Autodesk Inventor part; units mm, degrees
(part 6 of 6)
sketch "Sketch77" plane through (-67.6485, -56.3001, 10) normal (0, 0, -1) x (-1, 0, 0)
  line L0 (26.7044, 28.81) -> (18.3959, 20.5015)
  arc A0 (17.4062, 16.708) -> (18.3959, 20.5015) centre (3.9071, 22.2557) ccw
  line L1 (17.4062, 16.708) -> (10.5397, 0)
  line L2 (10.5397, 0) -> (0, 0)
  line L3 (0, 0) -> (0, -30)
  line L4 (0, -30) -> (10.5397, -30)
  line L5 (10.5397, -30) -> (17.4062, -46.708)
  arc A1 (18.3959, -50.5015) -> (17.4062, -46.708) centre (3.9071, -52.2557) ccw
  line L6 (18.3959, -50.5015) -> (26.7044, -58.81)
  line L7 (8.6997, -15) -> (26.7044, -58.81)
  line L8 (26.7044, 28.81) -> (8.6997, -15)
  line L9 (8.034, -77.4804) -> (-6.8327, -62.6138)
  line L10 (-6.8327, -62.6138) -> (-8.2078, -61.6851)
  line L11 (-8.2078, -61.6851) -> (-8.5835, -61.4603)
  line L12 (-8.5835, -61.4603) -> (-27.5835, -51.4603)
  line L13 (-27.5835, -51.4603) -> (-31.3094, -51.4603)
  line L14 (-31.3094, -51.4603) -> (-50.3094, -61.4603)
  line L15 (-50.3094, -61.4603) -> (-52.2336, -63.7126)
  line L16 (-52.2336, -63.7126) -> (-53.8304, -68.4099)
  arc A2 (-54.4465, -69.9343) -> (-53.8304, -68.4099) centre (-67.6485, -63.7126) ccw
  line L17 (-54.4465, -69.9343) -> (-54.4465, -82.65)
  line L18 (-48.4465, -65) -> (-54.4465, -82.65)
  line L19 (-29.4465, -55) -> (-48.4465, -65)
  line L20 (-10.4465, -65) -> (-29.4465, -55)
  line L21 (8.034, -77.4804) -> (-10.4465, -65)
  line L22 (-128.4643, -62.6138) -> (-143.3309, -77.4804)
  line L23 (-124.8505, -65) -> (-143.3309, -77.4804)
  line L24 (-105.8505, -55) -> (-124.8505, -65)
  line L25 (-86.8505, -65) -> (-105.8505, -55)
  line L26 (-80.8505, -82.65) -> (-86.8505, -65)
  line L27 (-80.8505, -82.65) -> (-80.8505, -69.9343)
  arc A3 (-81.4665, -68.4099) -> (-80.8505, -69.9343) centre (-67.6485, -63.7126) ccw
  line L28 (-81.4665, -68.4099) -> (-83.0633, -63.7126)
  line L29 (-83.0633, -63.7126) -> (-84.9875, -61.4603)
  line L30 (-84.9875, -61.4603) -> (-103.9875, -51.4603)
  line L31 (-103.9875, -51.4603) -> (-107.7134, -51.4603)
  line L32 (-107.7134, -51.4603) -> (-126.7134, -61.4603)
  line L33 (-126.7134, -61.4603) -> (-127.0891, -61.6851)
  line L34 (-127.0891, -61.6851) -> (-128.4643, -62.6138)
  line L35 (-50.3094, 31.4603) -> (-31.3094, 21.4603)
  line L36 (-6.8327, 32.6138) -> (8.034, 47.4804)
  line L37 (-10.4465, 35) -> (8.034, 47.4804)
  line L38 (-29.4465, 25) -> (-10.4465, 35)
  line L39 (-48.4465, 35) -> (-29.4465, 25)
  line L40 (-54.4465, 52.65) -> (-48.4465, 35)
  line L41 (-54.4465, 52.65) -> (-54.4465, 39.9343)
  arc A4 (-53.8304, 38.4099) -> (-54.4465, 39.9343) centre (-67.6485, 33.7126) ccw
  line L42 (-53.8304, 38.4099) -> (-52.2336, 33.7126)
  line L43 (-52.2336, 33.7126) -> (-50.3094, 31.4603)
  line L44 (-50.3094, 31.4603) -> (-31.3094, 21.4603)
  line L45 (-31.3094, 21.4603) -> (-27.5835, 21.4603)
  line L46 (-27.5835, 21.4603) -> (-8.5835, 31.4603)
  line L47 (-8.5835, 31.4603) -> (-8.2078, 31.6851)
  line L48 (-8.2078, 31.6851) -> (-6.8327, 32.6138)
  line L49 (-143.3309, 47.4804) -> (-128.4643, 32.6138)
  line L50 (-128.4643, 32.6138) -> (-127.0891, 31.6851)
  line L51 (-127.0891, 31.6851) -> (-126.7134, 31.4603)
  line L52 (-126.7134, 31.4603) -> (-107.7134, 21.4603)
  line L53 (-107.7134, 21.4603) -> (-103.9875, 21.4603)
  line L54 (-103.9875, 21.4603) -> (-84.9875, 31.4603)
  line L55 (-84.9875, 31.4603) -> (-83.0633, 33.7126)
  line L56 (-83.0633, 33.7126) -> (-81.4665, 38.4099)
  arc A5 (-80.8505, 39.9343) -> (-81.4665, 38.4099) centre (-67.6485, 33.7126) ccw
  line L57 (-80.8505, 39.9343) -> (-80.8505, 52.65)
  line L58 (-86.8505, 35) -> (-80.8505, 52.65)
  line L59 (-105.8505, 25) -> (-86.8505, 35)
  line L60 (-124.8505, 35) -> (-105.8505, 25)
  line L61 (-143.3309, 47.4804) -> (-124.8505, 35)
  line L62 (-162.0013, -58.81) -> (-155.7371, -52.5457)
  arc A6 (-155.2161, -49.5915) -> (-155.7371, -52.5457) centre (-141.1799, -53.5901) ccw
  line L63 (-155.2161, -49.5915) -> (-154.2755, -46.2898)
  line L64 (-154.2755, -46.2898) -> (-150.5441, -47.3528)
  line L65 (-150.5441, -47.3528) -> (-144.5534, -41.3621)
  line L66 (-144.5534, -41.3621) -> (-144.3898, -40.7877)
  line L67 (-144.3898, -40.7877) -> (-152.0837, -38.5959)
  line L68 (-152.0837, -38.5959) -> (-151.9306, -37.5)
  line L69 (-151.9306, -37.5) -> (-155.9306, -37.5)
  line L70 (-162.0013, -58.81) -> (-155.9306, -37.5)
  line L71 (-144.5534, 11.3621) -> (-150.5441, 17.3528)
  line L72 (-150.5441, 17.3528) -> (-154.2755, 16.2898)
  line L73 (-154.2755, 16.2898) -> (-155.2161, 19.5915)
  arc A7 (-155.7371, 22.5457) -> (-155.2161, 19.5915) centre (-141.1799, 23.5901) ccw
  line L74 (-155.7371, 22.5457) -> (-162.0013, 28.81)
  line L75 (-155.9306, 7.5) -> (-162.0013, 28.81)
  line L76 (-155.9306, 7.5) -> (-151.9306, 7.5)
  line L77 (-151.9306, 7.5) -> (-152.0837, 8.5959)
  line L78 (-152.0837, 8.5959) -> (-144.3898, 10.7877)
  line L79 (-144.3898, 10.7877) -> (-144.5534, 11.3621)
  arc A8 (26.7044, -58.81) -> (8.034, -77.4804) centre (40.2898, -91.0658) ccw
  arc A9 (-54.4465, -82.65) -> (-80.8505, -82.65) centre (-67.6485, -115.0647) ccw
  arc A10 (-143.3309, -77.4804) -> (-162.0013, -58.81) centre (-175.5867, -91.0658) ccw
  arc A11 (-162.0013, 28.81) -> (-143.3309, 47.4804) centre (-175.5867, 61.0658) ccw
  arc A12 (-80.8505, 52.65) -> (-54.4465, 52.65) centre (-67.6485, 85.0647) ccw
  arc A13 (8.034, 47.4804) -> (26.7044, 28.81) centre (40.2898, 61.0658) ccw
  line L80 (-54.4465, -82.65) -> (-80.8505, -82.65)
  line L81 (26.7044, -58.81) -> (8.034, -77.4804)
  line L82 (8.034, 47.4804) -> (26.7044, 28.81)
  line L83 (-80.8505, 52.65) -> (-54.4465, 52.65)
  line L84 (-162.0013, 28.81) -> (-143.3309, 47.4804)
  line L85 (-143.3309, -77.4804) -> (-162.0013, -58.81)
  point P0 (-67.6485, 56.3001)
extrude "Extrusion72" cut sketch "Sketch77" against normal blind 257.25 contours L85 A10 | L80 A9 | L81 A8 | A11 L84 | A12 L83 | A13 L82
body "Solid1"
